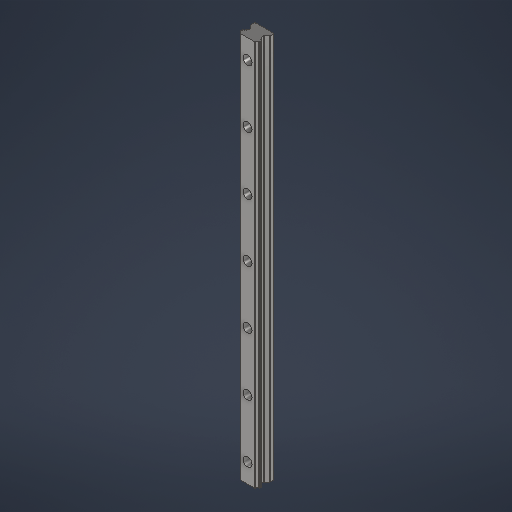
# Autodesk Inventor part: HGR20R-LinearRail300mm
Saved by Autodesk Inventor 2026.2 (Build 302298000, 298)
## iProperties
Created: 2026-06-17
Part Number: HGR20R-LinearRail300mm
Material: Stainless Steel
Document SubType Name: Modeling
Designer: Kenji
Density: 8 g/cm^3
Appearance: Semi-Polished
Author: Kenji
Autodesk Inventor part; units mm, degrees
ref_plane "YZ Plane" through (0, 0, 0) normal (1, 0, 0) x (0, 1, 0)
ref_plane "XZ Plane" through (0, 0, 0) normal (0, 1, 0) x (-1, 0, 0)
ref_plane "XY Plane" through (0, 0, 0) normal (0, 0, 1) x (1, 0, 0)
sketch "Sketch1" plane through (0, 0, 0) normal (0, 1, 0) x (-1, 0, 0)
  arc A0 (-9.8536, 6.1517) -> (-10, 5.7981) centre (-9.5, 5.7981) ccw
  line L0 (-10, 4.7409) -> (-10, 5.7981)
  arc A1 (-10, 4.7409) -> (-9.8536, 4.3873) centre (-9.5, 4.7409) ccw
  line L1 (-9.6906, 4.2244) -> (-9.8536, 4.3873)
  arc A2 (-9.6906, 4.2244) -> (-9.4318, 4.087) centre (-9.3371, 4.578) ccw
  arc A3 (-7.8468, 2.502) -> (-9.4318, 4.087) centre (-9.8106, 2.1232) ccw
  arc A4 (-7.8468, 2.502) -> (-7.6302, 2.1639) centre (-7.3529, 2.58) ccw
  line L2 (-6.8929, 1.4267) -> (-7.6302, 2.1639)
  arc A5 (-6.6, 0.7196) -> (-6.8929, 1.4267) centre (-7.6, 0.7196) ccw
  line L3 (-6.6, -0.8406) -> (-6.6, 0.7196)
  arc A6 (-6.8929, -1.5477) -> (-6.6, -0.8406) centre (-7.6, -0.8406) ccw
  line L4 (-9.7071, -4.3619) -> (-6.8929, -1.5477)
  arc A7 (-9.7071, -4.3619) -> (-10, -5.069) centre (-9, -5.069) ccw
  line L5 (-10, -7.7305) -> (-10, -5.069)
  line L6 (-9, -8.7305) -> (-10, -7.7305)
  line L7 (9, -8.7305) -> (-9, -8.7305)
  line L8 (10, -7.7305) -> (9, -8.7305)
  line L9 (10, -5.069) -> (10, -7.7305)
  arc A8 (10, -5.069) -> (9.7071, -4.3619) centre (9, -5.069) ccw
  line L10 (6.8929, -1.5477) -> (9.7071, -4.3619)
  arc A9 (6.6, -0.8406) -> (6.8929, -1.5477) centre (7.6, -0.8406) ccw
  line L11 (6.6, 0.7196) -> (6.6, -0.8406)
  arc A10 (6.8929, 1.4267) -> (6.6, 0.7196) centre (7.6, 0.7196) ccw
  line L12 (7.6302, 2.1639) -> (6.8929, 1.4267)
  arc A11 (7.6302, 2.1639) -> (7.8468, 2.502) centre (7.3529, 2.58) ccw
  arc A12 (9.4318, 4.087) -> (7.8468, 2.502) centre (9.8106, 2.1232) ccw
  arc A13 (9.4318, 4.087) -> (9.6906, 4.2244) centre (9.3371, 4.578) ccw
  line L13 (9.8536, 4.3873) -> (9.6906, 4.2244)
  arc A14 (9.8536, 4.3873) -> (10, 4.7409) centre (9.5, 4.7409) ccw
  line L14 (10, 5.7981) -> (10, 4.7409)
  arc A15 (10, 5.7981) -> (9.8536, 6.1517) centre (9.5, 5.7981) ccw
  line L15 (9.6906, 6.3146) -> (9.8536, 6.1517)
  arc A16 (9.6906, 6.3146) -> (9.4224, 6.4636) centre (9.3254, 5.9731) ccw
  arc A17 (7.8482, 8.0375) -> (9.4224, 6.4636) centre (9.8101, 8.4256) ccw
  arc A18 (7.8482, 8.0375) -> (7.6325, 8.3727) centre (7.3547, 7.957) ccw
  line L16 (7.2357, 8.7695) -> (7.6325, 8.3727)
  line L17 (-7.2357, 8.7695) -> (7.2357, 8.7695)
  line L18 (-7.6325, 8.3727) -> (-7.2357, 8.7695)
  arc A19 (-7.6325, 8.3727) -> (-7.8482, 8.0375) centre (-7.3547, 7.957) ccw
  arc A20 (-9.4224, 6.4636) -> (-7.8482, 8.0375) centre (-9.8101, 8.4256) ccw
  arc A21 (-9.4224, 6.4636) -> (-9.6906, 6.3146) centre (-9.3254, 5.9731) ccw
  line L19 (-9.8536, 6.1517) -> (-9.6906, 6.3146)
  point P0 (0, 0)
  point P1 (0, 5.2695)
  constraints: 44 point on circle, 40 end point, 22 centre point, 6 vertical, 2 horizontal, 100 other
extrude "Extrusion1" add sketch "Sketch1" along normal blind 400
sketch "Sketch2" plane through (-7.2357, 0, 8.7695) normal (0, 0, 1) x (1, 0, 0)
  circle A0 centre (7.2357, 20) radius 3
  line L0 (0, 0) -> (14.4714, 0) projected
  circle A1 centre (7.2357, 80) radius 3
  circle A2 centre (7.2357, 140) radius 3
  circle A3 centre (7.2357, 200) radius 3
  circle A4 centre (7.2357, 260) radius 3
  circle A5 centre (7.2357, 320) radius 3
  circle A6 centre (7.2357, 380) radius 3
  point P0 (7.2357, 0)
  point P1 (7.2357, 0)
  dimension "d2" = 6
  dimension "d3" = 20
  dimension "d4" = 60
  dimension "d5" = 60
  dimension "d6" = 60
  dimension "d7" = 60
  dimension "d13" = 60
  dimension "d14" = 60
  constraints: 7 centre point, 7 vertical alignment, 6 equal radius, 1 midpoint
  measures "d2" diameter of A0
  measures "d3" distance from line of A0.centre L0
  measures "d4" distance of A1.centre A0.centre
  measures "d5" distance of A2.centre A1.centre
  measures "d6" distance of A3.centre A2.centre
  measures "d7" distance of A4.centre A3.centre
  measures "d13" distance of A5.centre A4.centre
  measures "d14" distance of A6.centre A5.centre
extrude "Extrusion2" cut sketch "Sketch2" against normal through all contours A0 | A1 | A2 | A3 | A4
sketch "Sketch3" plane through (-7.2357, 0, 8.7695) normal (0, 0, 1) x (1, 0, 0)
  circle A0 centre (7.2357, 140) radius 3 projected
  circle A1 centre (7.2357, 80) radius 3 projected
  circle A2 centre (7.2357, 200) radius 3 projected
  circle A3 centre (7.2357, 20) radius 3 projected
  circle A4 centre (7.2357, 260) radius 3 projected
  line L0 (0, 0) -> (14.4714, 0) projected
  line L1 (14.4714, 0) -> (14.4714, 400) projected
  line L2 (0, 400) -> (14.4714, 400) projected
  line L3 (0, 0) -> (0, 400) projected
  circle A5 centre (7.2357, 20) radius 4.75
  circle A6 centre (7.2357, 80) radius 4.75
  circle A7 centre (7.2357, 140) radius 4.75
  circle A8 centre (7.2357, 200) radius 4.75
  circle A9 centre (7.2357, 260) radius 4.75
  circle A10 centre (7.2357, 320) radius 4.75
  circle A11 centre (7.2357, 380) radius 4.75
  point P0 (7.2357, 0)
  dimension "d10" = 9.5
  dimension "d17" = 60
  dimension "d18" = 60
  constraints: 7 centre point, 6 equal radius, 5 coincident, 2 vertical alignment
  measures "d10" diameter of A5
  measures "d17" distance of A10.centre A4.centre
  measures "d18" distance of A11.centre A10.centre
extrude "Extrusion3" cut sketch "Sketch3" against normal blind 8.4 contours A1 | A5 | A6 | A7 | A8 | A9
extrude "Extrusion4" cut sketch "Sketch2" against normal through all contours A5 | A6
extrude "Extrusion5" cut sketch "Sketch3" against normal up to surface (8.4 mm away) contours A10 | A11
equation "\"d5\" = d4"
equation "\"d6\" = d5"
equation "\"d7\" = d6"
equation "\"d13\" = d7"
equation "\"d14\" = d13"
equation "\"d18\" = d17"
body "Solid1"
